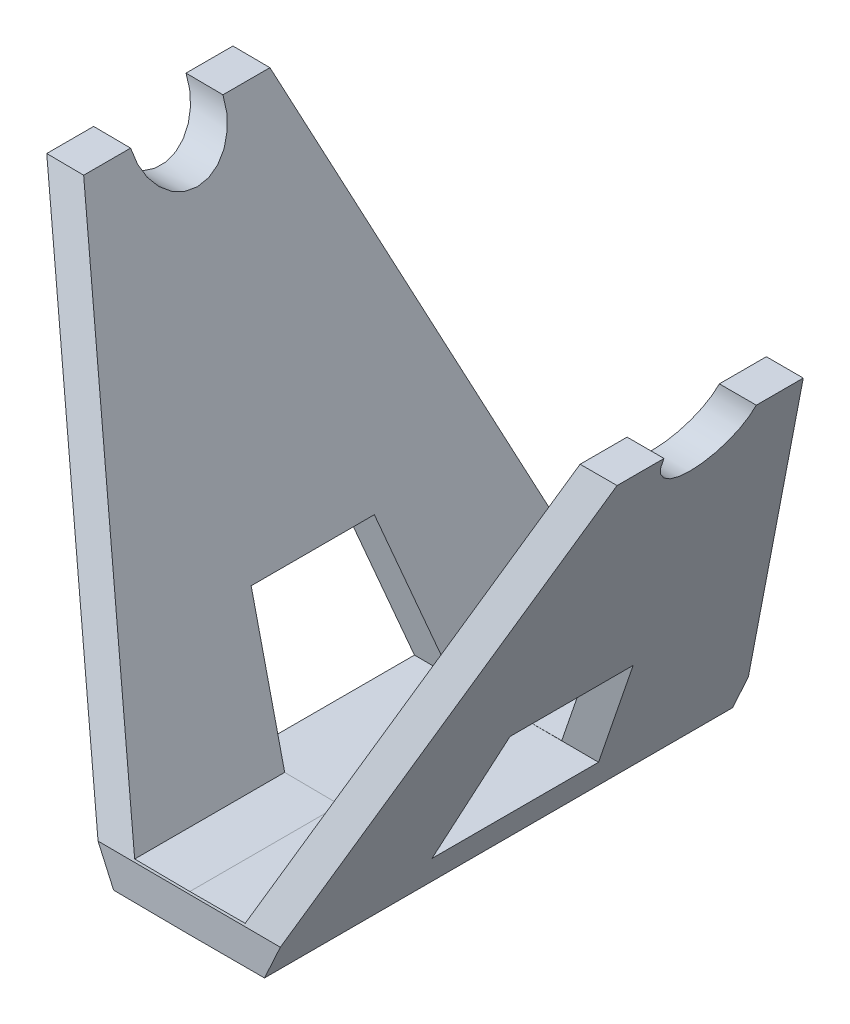
# Autodesk Inventor part: Shaft Bracket
Saved by Autodesk Inventor 2025 (Build 290162000, 162)
## iProperties
Created: 2024-06-10
Part Number: Shaft Bracket
Material: 일반
Document SubType Name: Modeling
Designer: unney
Density: 1 g/cm^3
Appearance: 기본값
Author: unney
Autodesk Inventor part; units mm, degrees
ref_plane "YZ Plane" through (0, 0, 0) normal (1, 0, 0) x (0, 1, 0)
ref_plane "XZ Plane" through (0, 0, 0) normal (0, 1, 0) x (-1, 0, 0)
ref_plane "XY Plane" through (0, 0, 0) normal (0, 0, 1) x (1, 0, 0)
sketch "스케치1" plane through (0, 0, 0) normal (0, 0, 1) x (1, 0, 0)
  line L0 (0, -5.830918) -> (0, 0.169082)
  line L1 (0, 0.169082) -> (9, 0.169082)
  line L2 (9, 0.169082) -> (40.62487, 69.169082)
  line L3 (40.62487, 69.169082) -> (46.62487, 69.169082)
  line L4 (46.62487, 69.169082) -> (46.62487, -5.830918)
  line L5 (46.62487, -5.830918) -> (0, -5.830918)
  line L6 (0.101104, 18.171631) -> (-0.081747, -25.238051)
  line L7 (0.050546, 0.168869) -> (-8.949135, 0.244688)
  line L8 (-8.949135, 0.244688) -> (-39.991604, 69.508658)
  line L9 (-45.991391, 69.559204) -> (-46.623216, -5.438135)
  line L10 (-46.623216, -5.438135) -> (0, -5.830918)
  line L11 (-39.991604, 69.508658) -> (-45.991391, 69.559204)
  point P0 (0, 0)
  point P1 (0, -2.830918)
  point P2 (0.025273, 0.169082)
  dimension "d1" = 9
  dimension "d2" = 6
  dimension "d6" = 75
  dimension "d10" = 6
  constraints: 24 end point, 5 symmetric about line, 3 perpendicular, 1 horizontal, 1 midpoint, 1 other
  measures "d1" distance of L0.end L1.end
  measures "d2" distance of L0.start L0.end
  measures "d6" distance of L3.end L4.end
  measures "d10" distance of L2.end L3.end
extrude "돌출1" add sketch "스케치1" along normal mid plane 80
sketch "스케치7" plane through (0, 0, 40) normal (0, 0, 1) x (1, 0, 0)
  line L0 (46.62487, 69.169082) -> (12.250011, -5.830918)
  line L1 (0, -5.830918) -> (46.62487, -5.830918)
  line L2 (40.62487, 69.169082) -> (9, 0.169082)
  line L3 (-46.623216, -5.438135) -> (-45.991391, 69.559204)
  line L4 (-45.991391, 69.559204) -> (-12.249577, -5.72772)
  line L5 (-46.623216, -5.438135) -> (0, -5.830918)
  line L6 (-8.949135, 0.244688) -> (-39.991604, 69.508658)
  line L7 (-45.991391, 69.559204) -> (-39.991604, 69.508658)
  line L8 (-45.991391, 69.559204) -> (-39.991604, 69.508658)
  line L9 (-45.991391, 69.559204) -> (-39.991604, 69.508658)
  line L10 (0.025273, 0.169082) -> (-8.949135, 0.244688)
  line L11 (-8.949135, 0.244688) -> (9, 0.169082)
  line L12 (40.62487, 69.169082) -> (46.62487, 69.169082)
  line L13 (46.62487, 69.169082) -> (46.62487, -5.830918)
  point P0 (0, 0)
  constraints: 14 end point, 2 collinear, 2 parallel, 2 point on line, 1 vertical
extrude "Side Cut" cut sketch "스케치7" against normal blind 80 contours L13 L1 L0 | L5 L3 L4
ref_plane "작업 평면2" through (46.62487, 11063.071025, -40) normal (-0.9999911, 0.0042122, 0) x (0, 0, 1)
sketch "스케치10" plane through (46.62487, 11063.071025, -40) normal (-0.9999911, 0.0042122, 0) x (0, 0, 1)
  line L0 (0, -11063.000086) -> (80, -11063.000086)
  line L1 (80, -11063.000086) -> (52.499992, -10979.461398)
  line L2 (27.499992, -10979.461398) -> (0, -11063.000086)
  line L3 (52.499992, -10979.461398) -> (27.499992, -10979.461398)
  line L4 (27.499992, -10979.461398) -> (0, -10979.461398)
  line L5 (0, -10979.461398) -> (0, -11063.000086)
  line L6 (52.499992, -10979.461398) -> (80, -10979.461398)
  line L7 (80, -10979.461398) -> (80, -11063.169273)
  point P0 (40, -11063.169273)
  point P1 (80, -11063.000086)
  dimension "d15" = 25
  constraints: 14 end point, 3 horizontal, 2 perpendicular
  measures "d15" distance of L1.end L2.start
extrude "Side cut 2" cut sketch "스케치10" along normal through all both and the other way through all contours L5 L4 L2 | L1 L6 L7
sketch "스케치13" plane through (0, 0, 0) normal (0, 0, 1) x (1, 0, 0)
  line L0 (-39.991604, 69.508658) -> (18.837539, 69.508658)
  line L1 (-8.949135, 0.244688) -> (-39.991604, 69.508658)
  line L2 (-39.991604, 69.508658) -> (-39.991604, -4.811798)
  point P0 (0, 0)
  constraints: 4 end point, 1 horizontal, 1 vertical
sketch "스케치14" plane through (-12.249577, -5.72772, -40) normal (-0.9125432, -0.4089802, 0) x (0, 0, 1)
  point P0 (40, 0.216957)
sketch "스케치15" plane through (0, 0, 0) normal (1, 0, 0) x (0, 1, 0)
  line L0 (69.508658, -17.229885) -> (69.508658, 17.229873)
  circle A0 centre (69.508658, -0.000006) radius 7.5
  point P0 (0, 0)
  dimension "d22" = 15
  constraints: 1 centre point, 1 midpoint
  measures "d22" diameter of A0
extrude "돌출4" cut sketch "스케치15" along normal mid plane 500
sketch "스케치16" plane through (-12.249577, -5.72772, -40) normal (-0.9125432, -0.4089802, 0) x (0, 0, 1)
  line L0 (80, -0.271818) -> (80, 64.330494)
  line L1 (0, 0.360915) -> (80, 0.360915)
  line L2 (5.851759, 10.460739) -> (70.884901, 10.460739)
  point P0 (40, 0.216957)
  point P1 (80, 32.029338)
  constraints: 4 end point, 2 horizontal, 2 vertical, 1 midpoint
offset faces "크기1" outward -2 faces at (34.073629, 46.148097, 24.817142) (9.082143, -1.851903, 40) (-33.634531, 46.4333, 24.817142)
offset faces "크기2" outward -2 faces at (34.073629, 46.148097, -24.81715) (9.082143, -1.851903, -40) (-33.634531, 46.4333, -24.81715)
sketch "스케치17" plane through (46.62487, 11063.071025, -40) normal (-0.9999911, 0.0042122, 0) x (0, 0, 1)
  line L0 (0, -11063.000086) -> (80, -11063.000086)
  line L1 (26.47346, -11063.000086) -> (53.52654, -11063.000086)
  line L2 (53.52654, -11063.000086) -> (50, -11043.000086)
  line L3 (50, -11043.000086) -> (30, -11043.000086)
  line L4 (30, -11043.000086) -> (26.47346, -11063.000086)
  line L5 (80, -11063.000086) -> (79.987556, -11062.962283)
  line L6 (79.987556, -11062.962283) -> (79.987556, -11006.10563)
  line L7 (40, -11063.169273) -> (40, -11000.137854)
  dimension "d28" = 10
  dimension "d29" = 20
  dimension "d30" = 20
  dimension "d31" = 100
  dimension "d32" = 100
  constraints: 12 end point, 2 point on line, 2 vertical, 1 parallel
  measures "d28" distance from line of L2.end L7
  measures "d29" distance between parallel lines of L0 L3
  measures "d30" distance of L2.end L3.end
  measures "d31" angle of L0 L2
  measures "d32" angle of L3 L4
extrude "돌출5" cut sketch "스케치17" along normal through all both and the other way through all
